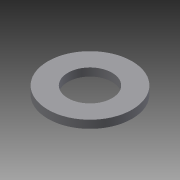
# Autodesk Inventor part: washer
Saved by Autodesk Inventor 2014 (Build 180170000, 170)
## iProperties
Created: 2013-07-23
Part Number: washer
Material: Generic
Document SubType Name: Modeling
Designer: employee
Density: 1 g/cm^3
Mass: 0.218466 g
Surface Area: 4.06271 cm^2
Volume: 0.218466 cm^3
Appearance: Default
Author: employee
Autodesk Inventor part; units mm, degrees
ref_plane "YZ Plane" through (0, 0, 0) normal (1, 0, 0) x (0, 1, 0)
ref_plane "XZ Plane" through (0, 0, 0) normal (0, 1, 0) x (-1, 0, 0)
ref_plane "XY Plane" through (0, 0, 0) normal (0, 0, 1) x (1, 0, 0)
sketch "Sketch1" plane through (0, 0, 0) normal (0, 0, 1) x (1, 0, 0)
  circle A0 centre (0, 0) radius 4.2
  circle A1 centre (0, 0) radius 8
  dimension "d0" = 8.4
  dimension "d2" = 16
  constraints: 2 centre point, 2 coincident
  measures "d0" diameter of A0
  measures "d2" diameter of A1
extrude "Extrusion1" add sketch "Sketch1" along normal blind 1.5
body "Solid1"
